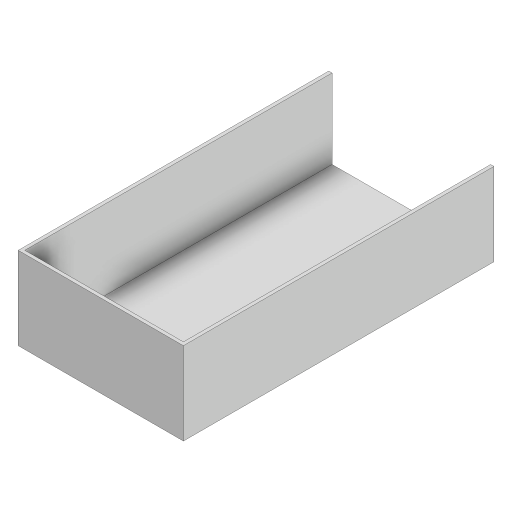
# Autodesk Inventor part: aaaa
Saved by Autodesk Inventor 2024.3 (Build 283343000, 343)
## iProperties
Created: 2025-09-24
Part Number: aaaa
Material: Generic
Document SubType Name: Modeling
Designer: danie
Density: 1 g/cm^3
Appearance: Default
Author: danie
Autodesk Inventor part; units mm, degrees
ref_plane "YZ Plane" through (0, 0, 0) normal (1, 0, 0) x (0, 1, 0)
ref_plane "XZ Plane" through (0, 0, 0) normal (0, 1, 0) x (-1, 0, 0)
ref_plane "XY Plane" through (0, 0, 0) normal (0, 0, 1) x (1, 0, 0)
sketch "Sketch1" plane through (0, 0, 0) normal (0, 1, 0) x (-1, 0, 0)
  line L0 (0, 0) -> (110, 0)
  line L1 (110, 0) -> (110, -200)
  line L2 (110, -200) -> (0, -200)
  line L3 (0, -200) -> (0, 0)
  line L4 (110, -200) -> (105, -200)
  line L5 (0, -200) -> (5, -200)
  line L6 (5, -200) -> (5, -10)
  line L7 (5, -10) -> (107.5, -10)
  line L8 (105, -200) -> (105, -10)
  line L9 (5, -200) -> (7, -200)
  line L10 (7, -200) -> (7, -12)
  line L11 (7, -12) -> (103, -12)
  line L12 (7, -200) -> (7, -198)
  line L13 (7, -198) -> (103, -198)
  line L14 (103, -198) -> (103, -12)
  line L15 (103, -198) -> (105, -198)
  dimension "d0" = 110
  dimension "d1" = 200
  dimension "d2" = 5
  dimension "d3" = 5
  dimension "d4" = 190
  dimension "d5" = 2
  dimension "d6" = 188
  dimension "d7" = 96
  dimension "d8" = 2
  constraints: 32 end point, 6 perpendicular, 6 point on line, 4 parallel, 1 horizontal, 1 vertical
  measures "d0" distance of L1.end L2.end
  measures "d1" distance of L0.end L1.end
  measures "d2" distance of L1.end L4.end
  measures "d3" distance of L2.end L5.end
  measures "d4" distance of L5.end L6.end
  measures "d5" distance of L5.end L9.end
  measures "d6" distance of L9.end L10.end
  measures "d7" distance of L10.end L11.end
  measures "d8" distance of L9.end L12.end
extrude "Extrusion1" add sketch "Sketch1" along normal blind 50 contours L6 L7 L8 L15 L14 L11 L10 L2
sketch "Sketch2" plane through (0, 0, 0) normal (0, -1, 0) x (1, 0, 0)
  line L0 (-5, -10) -> (-5, -200) projected
  line L1 (-5, -10) -> (-105.1065, -10)
  line L2 (-105.1065, -10) -> (-105.1065, -198)
  line L3 (-105.1065, -198) -> (-5, -198)
  line L4 (-5, -198) -> (-5, -10)
  point P0 (0, 0)
  constraints: 8 end point, 2 parallel, 1 horizontal, 1 perpendicular
extrude "Extrusion2" add sketch "Sketch2" against normal blind 2
sketch "Sketch3" plane through (-7, 0, -200) normal (-1, 0, 0) x (0, 0, 1)
  line L0 (190, 50) -> (0, 50) projected
  line L1 (0, 0) -> (2, 0)
  line L2 (2, 0) -> (2, 50)
  line L3 (2, 50) -> (0, 50)
  line L4 (0, 50) -> (0, 0)
  point P0 (200, 0)
  dimension "d13" = 2
  constraints: 8 end point, 2 parallel, 1 horizontal, 1 perpendicular, 1 point on line
  measures "d13" distance of L3.end L2.end
extrude "Extrusion3" cut sketch "Sketch3" against normal blind 23.25
body "Solid1"
